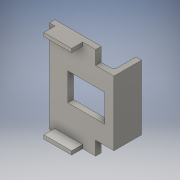
# Autodesk Inventor part: Ultrasonic
Saved by Autodesk Inventor 2016 (Build 200138000, 138)
## iProperties
Created: 2017-11-30
Part Number: Ultrasonic
Material: Stahl, Guss
Document SubType Name: Modeling
Designer: Chris
Density: 7.85 g/cm^3
Appearance: Halbpoliert
Mass: 43.8525 g
Surface Area: 45.2137 cm^2
Volume: 5.5863 cm^3
Author: Chris
Autodesk Inventor part; units mm, degrees
ref_plane "YZ Plane" through (0, 0, 0) normal (1, 0, 0) x (0, 1, 0)
ref_plane "XZ Plane" through (0, 0, 0) normal (0, 1, 0) x (-1, 0, 0)
ref_plane "XY Plane" through (0, 0, 0) normal (0, 0, 1) x (1, 0, 0)
sketch "Skizze1" plane through (0, 0, 0) normal (0, 1, 0) x (-1, 0, 0)
  line L0 (0, 0) -> (25, 0)
  line L1 (25, 0) -> (25, 50)
  line L2 (25, 50) -> (0, 50)
  line L3 (0, 42.5) -> (-9.9167, 42.5)
  line L4 (-9.9167, 42.5) -> (-9.9167, 7.5)
  line L5 (-9.9167, 7.5) -> (0, 7.5)
  line L6 (15, 32.5) -> (-5, 32.5)
  line L7 (-5, 32.5) -> (-5, 17.5)
  line L8 (-5, 17.5) -> (15, 17.5)
  line L9 (15, 17.5) -> (15, 32.5)
  line L10 (0, 7.5) -> (0, 17.5)
  line L11 (0, 32.5) -> (0, 42.5)
  line L12 (0, 50) -> (0, 32.5)
  line L13 (0, 17.5) -> (0, 0)
  dimension "d0" = 50
  dimension "d1" = 25
  dimension "d2" = 7.5
  dimension "d4" = 35
  dimension "d5" = 10
  dimension "d6" = 15
  dimension "d8" = 20
  dimension "d9" = 15
  constraints: 28 end point, 8 parallel, 3 horizontal, 3 perpendicular, 3 point on line
  measures "d0" distance of L0.end L1.end
  measures "d1" distance of L1.end L2.end
  measures "d2" distance between parallel lines of L2 L3
  measures "d4" distance of L3.end L4.end
  measures "d5" distance between parallel lines of L3 L6
  measures "d6" distance of L8.end L6.start
  measures "d8" distance of L7.end L8.end
  measures "d9" distance between parallel lines of L11 L9
extrude "Extrusion1" add sketch "Skizze1" along normal blind 3 contours L13 L10 L8 L9 L6 L11 L12 L2 L1 L0 | L5 L4 L3 L11 L6 L7 L8 L10
sketch "Skizze2" plane through (0, 0, 42.5) normal (0, 0, 1) x (1, 0, 0)
  line L0 (9.9167, 0) -> (9.9167, 3) projected
  line L1 (9.9167, 3) -> (6.9167, 3)
  line L2 (6.9167, 3) -> (6.9167, 15)
  line L3 (6.9167, 15) -> (9.9167, 15)
  line L4 (9.9167, 15) -> (9.9167, 3)
  point P0 (0, 0)
  dimension "d12" = 3
  dimension "d13" = 12
  constraints: 8 end point, 2 parallel, 1 horizontal, 1 perpendicular
  measures "d12" distance of L2.end L3.end
  measures "d13" distance of L1.end L2.end
extrude "Extrusion2" add sketch "Skizze2" against normal up to surface (35 mm away)
fillet "Rundung1" radius 2 1 edges at (6.9167, 3, 25)
sketch "Skizze3" plane through (0, 0, 0) normal (0, -1, 0) x (1, 0, 0)
  line L0 (-22, 0) -> (-7, 0)
  line L1 (-7, 0) -> (-7, 2)
  line L2 (-7, 2) -> (-22, 2)
  line L3 (-22, 2) -> (-22, 0)
  line L4 (-22, 48) -> (-7, 48)
  line L5 (-7, 48) -> (-7, 50)
  line L6 (-7, 50) -> (-22, 50)
  line L7 (-22, 50) -> (-22, 48)
  line L8 (-25, 50) -> (0, 50) projected
  line L9 (0, 50) -> (0, 42.5) projected
  point P0 (0, 0)
  dimension "d17" = 2
  dimension "d18" = 2
  dimension "d19" = 46
  dimension "d20" = 15
  dimension "d21" = 15
  dimension "d22" = 0
  dimension "d23" = 7
  constraints: 16 end point, 4 parallel, 2 horizontal, 2 perpendicular, 1 point on line
  measures "d17" distance between parallel lines of L0 L2
  measures "d18" distance of L6.end L4.start
  measures "d19" distance between parallel lines of L4 L2
  measures "d20" distance of L1.end L2.end
  measures "d21" distance of L5.end L6.end
  measures "d22" distance between parallel lines of L8 L6
  measures "d23" distance between parallel lines of L9 L5
extrude "Extrusion3" add sketch "Skizze3" along normal blind 6
